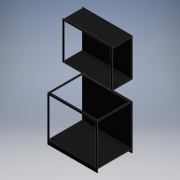
# Autodesk Inventor part: esqueleto_mueble
Saved by Autodesk Inventor 2016 (Build 200138000, 138)
## iProperties
Created: 2015-11-24
Part Number: esqueleto_mueble
Material: Generic
Document SubType Name: Modeling
Designer: Daniela
Density: 1 g/cm^3
Appearance: Glossy - Black
Author: Daniela
Autodesk Inventor part; units mm, degrees
ref_plane "YZ Plane" through (0, 0, 0) normal (1, 0, 0) x (0, 1, 0)
ref_plane "XZ Plane" through (0, 0, 0) normal (0, 1, 0) x (-1, 0, 0)
ref_plane "XY Plane" through (0, 0, 0) normal (0, 0, 1) x (1, 0, 0)
sketch "Sketch1" plane through (0, 0, 0) normal (0, 0, 1) x (1, 0, 0)
  line L0 (0, 0) -> (1483.3333, 0)
  line L1 (1483.3333, 0) -> (1483.3333, 10)
  line L2 (1483.3333, 10) -> (0, 10)
  line L3 (0, 10) -> (0, 0)
  dimension "ancho" = 1483.3333
  dimension "espesor" = 10
  constraints: 8 end point, 2 parallel, 1 horizontal, 1 perpendicular
  measures "ancho" distance of L1.end L2.end
  measures "espesor" distance of L0.end L1.end
extrude "Extrusion1" add sketch "Sketch1" along normal blind 900
sketch "Sketch2" plane through (0, 0, 0) normal (0, -1, 0) x (1, 0, 0)
  line L0 (0, 0) -> (1483.3333, 0) construction
  line L1 (1483.3333, 0) -> (1483.3333, 900) construction
  line L2 (0, 900) -> (1483.3333, 900) construction
  line L3 (0, 0) -> (0, 900) construction
  line L4 (0, 0) -> (0, 900) projected
  line L5 (0, 70) -> (1483.3333, 70)
  line L6 (1483.3333, 70) -> (1483.3333, 80)
  line L7 (1483.3333, 80) -> (0, 80)
  line L8 (0, 80) -> (0, 70)
  line L9 (0, 900) -> (1483.3333, 900) projected
  line L10 (1483.3333, 0) -> (1483.3333, 900) projected
  line L11 (0, 900) -> (1483.3333, 900)
  line L12 (1483.3333, 900) -> (1483.3333, 890)
  line L13 (1483.3333, 890) -> (0, 890)
  line L14 (0, 890) -> (0, 900)
  dimension "d5" = 10
  dimension "d6" = 10
  dimension "d7" = 80
  constraints: 16 end point, 4 parallel, 3 point on line, 2 horizontal, 2 perpendicular
  measures "d5" distance between parallel lines of L5 L7
  measures "d6" distance between parallel lines of L2 L13
  measures "d7" distance between parallel lines of L0 L7
extrude "Extrusion2" add sketch "Sketch2" along normal blind 690 contours L4 L7 L6 L5 | L4 L9 L10 L13
sketch "Sketch3" plane through (0, 0, 900) normal (0, 0, 1) x (1, 0, 0)
  line L0 (1483.3333, 10) -> (1483.3333, -690) projected
  line L1 (1483.3333, 10) -> (0, 10) projected
  line L2 (0, 10) -> (0, -690) projected
  line L3 (1483.3333, -690) -> (0, -690) projected
  line L4 (30, -660) -> (30, -20)
  line L5 (30, -20) -> (1453.3333, -20)
  line L6 (1453.3333, -20) -> (1453.3333, -660)
  line L7 (1453.3333, -660) -> (30, -660)
  point P0 (0, 0)
  dimension "d10" = 30
  constraints: 8 end point, 3 other
  measures "d10" distance between parallel lines of L1 L5
extrude "Extrusion3" cut sketch "Sketch3" against normal up to next contours L4 L5 L6 L7
sketch "Sketch4" plane through (0, -690, 0) normal (0, -1, 0) x (1, 0, 0)
  line L0 (0, 70) -> (1483.3333, 70) construction
  line L1 (1483.3333, 70) -> (1483.3333, 80) construction
  line L2 (1483.3333, 80) -> (0, 80) construction
  line L3 (0, 80) -> (0, 70) construction
  line L4 (0, 900) -> (0, 890) construction
  line L5 (0, 890) -> (1483.3333, 890) construction
  line L6 (1483.3333, 890) -> (1483.3333, 900) construction
  line L7 (1483.3333, 900) -> (0, 900) construction
  line L8 (1483.3333, 70) -> (0, 70) construction
  line L9 (0, 0) -> (0, 70) construction
  line L10 (0, 0) -> (1483.3333, 0) construction
  line L11 (1483.3333, 0) -> (1483.3333, 70) construction
  line L12 (0, 900) -> (1483.3333, 900)
  line L13 (1483.3333, 900) -> (1483.3333, 0)
  line L14 (1483.3333, 0) -> (0, 0)
  line L15 (0, 0) -> (0, 900)
  line L16 (1483.3333, 80) -> (0, 80) projected
  line L17 (30, 80) -> (1453.3333, 80)
  line L18 (1453.3333, 80) -> (1453.3333, 890)
  line L19 (1453.3333, 890) -> (30, 890)
  line L20 (30, 890) -> (30, 80)
  dimension "d13" = 30
  dimension "d14" = 30
  constraints: 16 end point, 4 parallel, 2 horizontal, 2 perpendicular, 2 point on line
  measures "d13" distance between parallel lines of L15 L20
  measures "d14" distance between parallel lines of L18 L13
extrude "Extrusion4" add sketch "Sketch4" against normal blind 10 contours L12 L13 L16 L18 L19 L20 L15 | L16 L13 L14 L15
ref_plane "Work Plane1" through (0, 0, 1280) normal (0, 0, 1) x (1, 0, 0)
sketch "Sketch5" plane through (0, 0, 1280) normal (0, 0, 1) x (1, 0, 0)
  line L0 (1483.3333, 10) -> (0, 10) projected
  line L1 (0, 10) -> (0, -690) projected
  line L2 (1483.3333, 10) -> (1483.3333, -690) projected
  line L3 (1483.3333, -690) -> (0, -690) projected
  line L4 (0, 10) -> (1483.3333, 10)
  line L5 (1483.3333, 10) -> (1483.3333, -390)
  line L6 (1483.3333, -390) -> (0, -390)
  line L7 (0, -390) -> (0, 10)
  line L8 (1453.3333, -660) -> (1453.3333, -20) projected
  line L9 (0, -390) -> (1453.3333, -390)
  line L10 (1453.3333, -390) -> (1453.3333, -380)
  line L11 (1453.3333, -380) -> (0, -380)
  line L12 (0, -380) -> (0, -390)
  point P0 (0, 0)
  dimension "d36" = 1483.3333
  dimension "profundidad2" = 400
  dimension "d39" = 10
  constraints: 16 end point, 4 parallel, 2 horizontal, 2 perpendicular, 1 point on line
  measures "d36" distance of L5.end L6.end
  measures "profundidad2" distance of L4.end L5.end
  measures "d39" distance between parallel lines of L6 L11
extrude "Extrusion5" add sketch "Sketch5" along normal blind 10 contours L2 L6 L8 L11 L1 L0 | L11 L8 L6 L1
sketch "Sketch9" plane through (0, -690, 0) normal (0, -1, 0) x (1, 0, 0)
  line L0 (30, 890) -> (1453.3333, 890) construction
  line L1 (1453.3333, 80) -> (30, 80) construction
  line L2 (0, 900) -> (0, 0) construction
  line L3 (1483.3333, 0) -> (0, 0) construction
  line L4 (1483.3333, 900) -> (1483.3333, 0) construction
  line L5 (1483.3333, 900) -> (0, 900) construction
  line L6 (1483.3333, 70) -> (1483.3333, 0) projected
  line L7 (0, 900) -> (1483.3333, 900)
  line L8 (1483.3333, 900) -> (1483.3333, 870)
  line L9 (1483.3333, 870) -> (0, 870)
  line L10 (0, 870) -> (0, 900)
  line L11 (1453.3333, 890) -> (1453.3333, 80) projected
  line L12 (30, 80) -> (30, 890) projected
  point P0 (1483.3333, 890)
  point P1 (1483.3333, 80)
  dimension "d32" = 30
  constraints: 8 end point, 2 parallel, 1 horizontal, 1 perpendicular, 1 point on line
  measures "d32" distance between parallel lines of L9 L5
extrude "Extrusion9" add sketch "Sketch9" against normal blind 10
sketch "Boceto10" plane through (0, 0, 1290) normal (0, 0, 1) x (1, 0, 0)
  line L0 (0, 10) -> (0, -390) projected
  line L1 (0, -390) -> (1483.3333, -390) projected
  line L2 (1483.3333, -390) -> (1483.3333, 10) projected
  line L3 (1483.3333, 10) -> (0, 10) projected
  line L4 (1483.3333, 10) -> (1483.3333, -690) projected
  line L5 (0, -390) -> (1483.3333, -390)
  line L6 (1483.3333, -390) -> (1483.3333, -380)
  line L7 (1483.3333, -380) -> (0, -380)
  line L8 (0, -380) -> (0, -390)
  line L9 (0, 10) -> (1483.3333, 10)
  line L10 (1483.3333, 10) -> (1483.3333, 0)
  line L11 (1483.3333, 0) -> (0, 0)
  line L12 (0, 0) -> (0, 10)
  point P0 (0, 0)
  dimension "d40" = 10
  dimension "d41" = 10
  constraints: 16 end point, 4 parallel, 2 horizontal, 2 perpendicular, 2 point on line
  measures "d40" distance between parallel lines of L3 L11
  measures "d41" distance between parallel lines of L1 L7
extrude "Extrusión10" add sketch "Boceto10" along normal blind 750 contours L3 L2 L11 L0 | L7 L2 L1 L0
sketch "Boceto11" plane through (0, -390, 1280) normal (0, -1, 0) x (1, 0, 0)
  line L0 (0, 760) -> (1483.3333, 760) projected
  line L1 (1483.3333, 0) -> (1483.3333, 760) projected
  line L2 (0, 760) -> (1483.3333, 760) projected
  line L3 (0, 0) -> (0, 760) projected
  line L4 (30, 730) -> (1453.3333, 730)
  line L5 (1453.3333, 730) -> (1453.3333, 10)
  line L6 (1453.3333, 10) -> (30, 10)
  line L7 (30, 10) -> (30, 730)
  line L8 (0, 0) -> (1483.3333, 0) projected
  point P0 (0, -1280)
  dimension "d44" = 30
  dimension "d45" = 30
  dimension "d46" = 30
  constraints: 8 end point, 2 parallel, 1 horizontal, 1 perpendicular
  measures "d44" distance between parallel lines of L3 L7
  measures "d45" distance between parallel lines of L1 L5
  measures "d46" distance between parallel lines of L0 L4
extrude "Extrusión11" cut sketch "Boceto11" against normal up to next contours L4 L5 L6 L7
sketch "Sketch13" plane through (1483.3333, -390, 1280) normal (1, 0, 0) x (0, 0, -1)
  line L0 (0, 0) -> (0, 400) construction
  line L1 (0, 400) -> (-760, 400) construction
  line L2 (-10, 390) -> (-760, 390) construction
  line L3 (-10, 10) -> (-760, 10) construction
  line L4 (-760, 0) -> (-760, 10) construction
  line L5 (0, 0) -> (-760, 0) construction
  line L6 (1280, 400) -> (-760, 400) projected
  line L7 (-740, 0) -> (-730, 0)
  line L8 (-730, 0) -> (-730, 400)
  line L9 (-730, 400) -> (-740, 400)
  line L10 (-740, 400) -> (-740, 0)
  line L11 (-760, 390) -> (-760, 400) projected
  line L12 (-10, 10) -> (-10, 390) projected
  point P0 (1280, 390)
  point P1 (1030, 400)
  dimension "d53" = 10
  dimension "d54" = 20
  constraints: 8 end point, 2 parallel, 2 point on line, 1 horizontal, 1 perpendicular
  measures "d53" distance between parallel lines of L8 L10
  measures "d54" distance between parallel lines of L10 L4
extrude "Extrusion13" add sketch "Sketch13" against normal blind 1483.3333
equation "\"d5\" = espesor"
equation "\"d6\" = espesor"
equation "\"d10\" = 3 * espesor"
equation "\"d13\" = 3 * espesor"
equation "\"d14\" = 3 * espesor"
equation "\"d15\" = espesor"
equation "\"d36\" = ancho"
equation "\"d39\" = espesor"
equation "\"d18\" = espesor"
equation "\"d32\" = 3 * espesor"
equation "\"d33\" = espesor"
equation "\"d40\" = espesor"
equation "\"d41\" = espesor"
equation "\"d44\" = 3 * espesor"
equation "\"d45\" = 3 * espesor"
equation "\"d46\" = 3 * espesor"
equation "\"d53\" = espesor"
equation "\"d54\" = 2 * espesor"
equation "\"d55\" = ancho"
body "Solid1"
